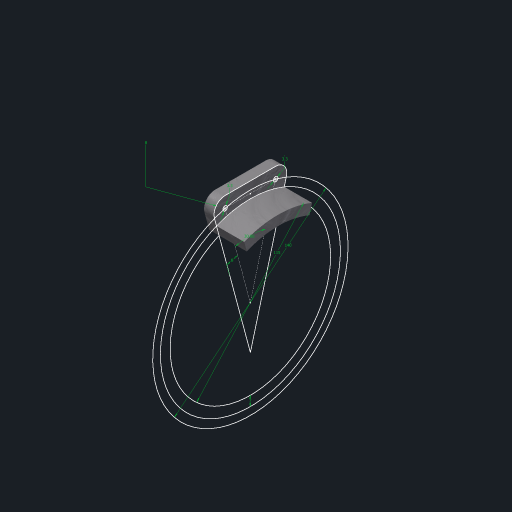
# Autodesk Inventor part: SEGURO_CANALETA
Saved by Autodesk Inventor 2024.3 (Build 283343000, 343)
## iProperties
Created: 2024-07-12
Part Number: SEGURO_CANALETA
Material: Steel, Mild, Welded
Document SubType Name: Modeling
Designer: Niler
Density: 7.85 g/cm^3
Appearance: Weld - Steel Mild
Author: Niler
Autodesk Inventor part; units mm, degrees
ref_plane "YZ Plane" through (0, 0, 0) normal (1, 0, 0) x (0, 1, 0)
ref_plane "XZ Plane" through (0, 0, 0) normal (0, 1, 0) x (-1, 0, 0)
ref_plane "XY Plane" through (0, 0, 0) normal (0, 0, 1) x (1, 0, 0)
sketch "Sketch1" plane through (0, 0, 0) normal (1, 0, 0) x (0, 1, 0)
  circle A0 centre (0, 0) radius 70
  line L0 (0, 0) -> (67.6148, 18.1173) construction
  line L1 (67.6148, -18.1173) -> (0, 0) construction
  line L2 (67.6148, -18.1173) -> (67.6148, 18.1173) construction
  circle A1 centre (67.6148, 18.1173) radius 1.65
  circle A2 centre (67.6148, -18.1173) radius 1.65
  circle A3 centre (0, 0) radius 57.5
  line L3 (65.5443, 25.8447) -> (-30.9096, 0)
  line L4 (-30.9096, 0) -> (65.5443, -25.8447)
  line L5 (75.6148, -18.1173) -> (75.6148, 18.1173)
  arc A4 (75.6148, 18.1173) -> (65.5443, 25.8447) centre (67.6148, 18.1173) ccw
  arc A5 (65.5443, -25.8447) -> (75.6148, -18.1173) centre (67.6148, -18.1173) ccw
  circle A6 centre (0, 0) radius 64.5
  point P0 (67.6148, 0)
  point P1 (52.93, 22.4648)
  point P2 (52.93, -22.4648)
  point P3 (59.7506, 24.2923)
  point P4 (59.7506, -24.2923)
  dimension "d0" = 140
  dimension "d1" = 30
  dimension "d2" = 3.3
  dimension "d3" = 3.3
  dimension "d4" = 115
  dimension "d5" = 8
  dimension "d6" = 8
  dimension "d7" = 7
  constraints: 12 end point, 7 centre point, 6 point on circle, 4 coincident, 4 tangent, 1 equal radius, 1 horizontal alignment, 1 midpoint, 1 vertical, 2 other
  measures "d0" diameter of A0
  measures "d1" angle of L0 L1
  measures "d2" diameter of A1
  measures "d3" diameter of A2
  measures "d4" diameter of A3
  measures "d5" distance between parallel lines of L0 L3
  measures "d6" radius of A4
  measures "d7" radial gap between concentric circles of A3 A6
extrude "Extrusion1" add sketch "Sketch1" against normal blind 7 contours A0 A2 L4 A6 L3 A1 | A0 A1 L3 A4 L5 A5 L4 A2 | A6 L4 A3 L3 picked at (61.9888, 2.7598)
extrude "Extrusion2" add sketch "Sketch1" along normal blind 20 contours A6 L4 A3 L3 picked at (61.9888, 2.7598)
body "Solid1"
